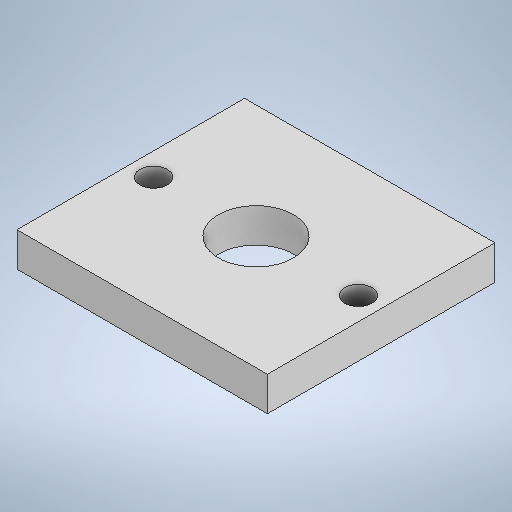
# Autodesk Inventor part: Taststift_Kappe
Saved by Autodesk Inventor 2025 (Build 290162000, 162)
## iProperties
Created: 2026-07-12
Part Number: Taststift_Kappe
Material: Generisch
Document SubType Name: Modeling
Designer: wavid
Mass: 1.19022 g
Surface Area: 11.5292 cm^2
Volume: 1.19022 cm^3
Density: 1 g/cm^3
Appearance: Vorgabe
Author: wavid
Autodesk Inventor part; units mm, degrees
ref_plane "YZ Plane" through (0, 0, 0) normal (1, 0, 0) x (0, 1, 0)
ref_plane "XZ Plane" through (0, 0, 0) normal (0, 1, 0) x (-1, 0, 0)
ref_plane "XY Plane" through (0, 0, 0) normal (0, 0, 1) x (1, 0, 0)
sketch "Skizze1" plane through (0, 0, 0) normal (0, 0, 1) x (1, 0, 0)
  line L0 (-11, -10) -> (11, -10)
  line L1 (11, -10) -> (11, 10)
  line L2 (11, 10) -> (-11, 10)
  line L3 (-11, 10) -> (-11, -10)
  constraints: 8 end point, 2 parallel, 1 horizontal, 1 perpendicular
extrude "Extrusion1" add sketch "Skizze1" along normal blind 3
sketch "Skizze2" plane through (0, 0, 0) normal (0, 0, 1) x (1, 0, 0)
  circle A0 centre (0, 0) radius 3.3
  constraints: 1 centre point
extrude "Extrusion2" cut sketch "Skizze2" along normal blind 3.2
sketch "Skizze3" plane through (0, 0, 0) normal (0, 0, 1) x (1, 0, 0)
  circle A0 centre (-9, 0) radius 1.2
  constraints: 1 centre point
extrude "Extrusion3" cut sketch "Skizze3" along normal blind 3.2
sketch "Skizze4" plane through (0, 0, 0) normal (0, 0, 1) x (1, 0, 0)
  circle A0 centre (9, 0) radius 1.2
  constraints: 1 centre point
extrude "Extrusion4" cut sketch "Skizze4" along normal blind 3.2
